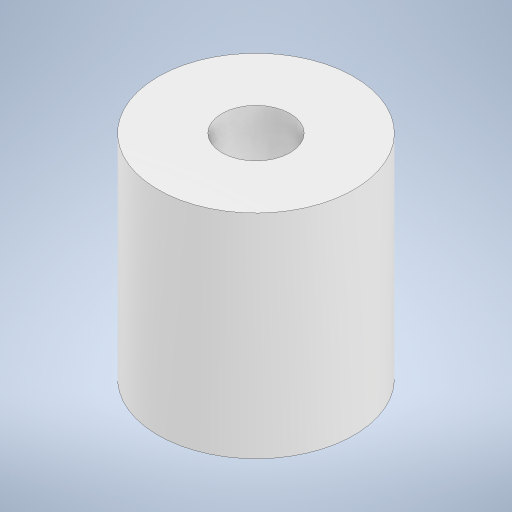
# Autodesk Inventor part: Spacer
Saved by Autodesk Inventor 2024 (Build 280153000, 153)
## iProperties
Created: 2023-04-24
Part Number: Spacer
Material: ABS Plastic
Document SubType Name: Modeling
Designer: byrne
Density: 1.06 g/cm^3
Appearance: Smooth - White
Author: byrne
Autodesk Inventor part; units mm, degrees
ref_plane "YZ Plane" through (0, 0, 0) normal (1, 0, 0) x (0, 1, 0)
ref_plane "XZ Plane" through (0, 0, 0) normal (0, 1, 0) x (-1, 0, 0)
ref_plane "XY Plane" through (0, 0, 0) normal (0, 0, 1) x (1, 0, 0)
sketch "Sketch1" plane through (0, 0, 0) normal (0, 1, 0) x (-1, 0, 0)
  circle A0 centre (0, 0) radius 2.54
  circle A1 centre (0, 0) radius 7.3025
  dimension "d0" = 5.08
  dimension "d1" = 4.7625
  constraints: 2 centre point, 1 coincident
  measures "d0" diameter of A0
  measures "d1" radial gap between concentric circles of A0 A1
extrude "Extrusion1" add sketch "Sketch1" along normal blind 15.875
body "Solid1"
